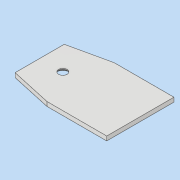
# Autodesk Inventor part: phototransistorMount2
Saved by Autodesk Inventor 2017 (Build 210142000, 142)
## iProperties
Created: 2016-12-12
Part Number: phototransistorMount2
Material: ABS Plastic
Document SubType Name: Modeling
Designer: techn
Density: 1.06 g/cm^3
Appearance: Smooth - White
Author: techn
Autodesk Inventor part; units mm, degrees
ref_plane "YZ Plane" through (0, 0, 0) normal (1, 0, 0) x (0, 1, 0)
ref_plane "XZ Plane" through (0, 0, 0) normal (0, 1, 0) x (-1, 0, 0)
ref_plane "XY Plane" through (0, 0, 0) normal (0, 0, 1) x (1, 0, 0)
sketch "Sketch1" plane through (0, 0, 0) normal (0, 1, 0) x (-1, 0, 0)
  line L0 (0, 0) -> (0, -11.938)
  line L1 (-15.24, 3.3655) -> (-15.24, -15.3035)
  line L2 (0, 0) -> (-15.24, 3.3655)
  line L3 (0, -11.938) -> (-15.24, -15.3035)
  line L4 (-15.24, 3.3655) -> (-19.05, 3.3655)
  line L5 (-19.05, 3.3655) -> (-19.05, 2.0955)
  line L6 (-19.05, 2.0955) -> (-15.24, 2.0955)
  line L7 (-15.24, 2.0955) -> (-15.24, 3.3655)
  line L8 (-15.24, -15.3035) -> (-19.05, -15.3035)
  line L9 (-19.05, -15.3035) -> (-19.05, -14.0335)
  line L10 (-19.05, -14.0335) -> (-15.24, -14.0335)
  line L11 (-15.24, -14.0335) -> (-15.24, -15.3035)
  line L12 (0, 0) -> (0, 3.175)
  line L13 (-15.24, 3.3655) -> (-15.24, 6.5405)
  line L14 (0, -11.938) -> (0, -15.113)
  line L15 (-15.24, -15.3035) -> (-15.24, -18.4785)
  line L16 (-15.24, -18.4785) -> (0, -15.113)
  line L17 (0, 3.175) -> (-15.24, 6.5405)
  line L18 (-15.24, 6.5405) -> (-34.29, 6.5405)
  line L19 (-19.05, 3.3655) -> (-34.29, 3.3655)
  line L20 (-34.29, 3.3655) -> (-34.29, 6.5405)
  line L21 (-15.24, -18.4785) -> (-34.29, -18.4785)
  line L22 (-34.29, -18.4785) -> (-34.29, -15.3035)
  line L23 (-34.29, -15.3035) -> (-19.05, -15.3035)
  line L24 (-34.29, 6.5405) -> (-37.465, 6.5405)
  line L25 (-37.465, 6.5405) -> (-37.465, -18.4785)
  line L26 (-37.465, -18.4785) -> (-34.29, -18.4785)
  line L27 (-34.29, -18.4785) -> (-34.29, 6.5405)
  line L28 (-15.24, -15.3035) -> (-34.29, -15.3035)
  line L29 (-34.29, -15.3035) -> (-34.29, 3.3655)
  line L30 (-34.29, 3.3655) -> (-15.24, 3.3655)
  line L31 (-15.24, 3.3655) -> (-15.24, -15.3035)
  line L32 (-15.24, 3.3655) -> (-34.29, 3.3655)
  line L33 (-34.29, 3.3655) -> (-34.29, 6.5405)
  line L34 (-34.29, 6.5405) -> (-15.24, 6.5405)
  line L35 (-15.24, 6.5405) -> (-15.24, 3.3655)
  dimension "d0" = 11.938
  dimension "d1" = 15.24
  dimension "d2" = 18.669
  dimension "d3" = 3.3655
  dimension "d4" = 3.81
  dimension "d5" = 1.27
  dimension "d6" = 3.81
  dimension "d7" = 1.27
  dimension "d8" = 3.175
  dimension "d9" = 3.175
  dimension "d10" = 3.175
  dimension "d11" = 3.175
  dimension "d12" = 19.05
  dimension "d13" = 3.175
  constraints: 72 end point, 11 parallel, 8 perpendicular, 6 horizontal, 6 vertical, 2 point on line
  measures "d0" distance of L0.start L0.end
  measures "d1" distance between parallel lines of L1 L0
  measures "d2" distance of L1.start L1.end
  measures "d3" vertical distance of L1.start L0.start
  measures "d4" distance of L6.end L5.end
  measures "d5" distance of L5.end L4.end
  measures "d6" distance of L9.end L10.end
  measures "d7" distance of L8.end L9.end
  measures "d8" distance of L0.start L12.end
  measures "d9" distance of L1.start L13.end
  measures "d10" distance of L0.end L14.end
  measures "d11" distance of L1.end L15.end
  measures "d12" distance of L13.end L18.end
  measures "d13" distance of L26.end L25.end
extrude "Extrusion4" add sketch "Sketch1" along normal blind 1.5875
sketch "Sketch4" plane through (0, 1.5875, 0) normal (0, 1, 0) x (1, 0, 0)
  circle A0 centre (8.636, 5.969) radius 1.5875
  line L0 (0, 15.113) -> (0, -3.175) projected
  point P0 (0, 0)
  dimension "d26" = 3.175
  dimension "d27" = 8.636
  constraints: 1 centre point
  measures "d26" diameter of A0
  measures "d27" distance from line of L0 A0.centre
extrude "Extrusion5" cut sketch "Sketch4" against normal blind 1.5875
chamfer "Chamfer2" distance 1.27 angle 45 1 edges at (7.0485, 0, -5.969)
equation "\"d3\" = -0.5 * d0 + 0.5 * d2"
body "Solid2"
